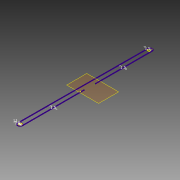
# Autodesk Inventor part: FDM20-BandaX-01
Saved by Autodesk Inventor 2015 (Build 190159000, 159)
## iProperties
Created: 2016-07-12
Part Number: FDM20-BandaX-01
Material: Generic
Document SubType Name: Modeling
Designer: Proyectil
Density: 1 g/cm^3
Appearance: Default
Author: Proyectil
Autodesk Inventor part; units mm, degrees
ref_plane "YZ Plane" through (0, 0, 0) normal (1, 0, 0) x (0, 1, 0)
ref_plane "XZ Plane" through (0, 0, 0) normal (0, 1, 0) x (-1, 0, 0)
ref_plane "XY Plane" through (0, 0, 0) normal (0, 0, 1) x (1, 0, 0)
ref_plane "Work Plane1" through (0.0298, -19.0597, 0) normal (0, 0, 1) x (1, -0.0002116, 0)
sketch "Sketch1" plane through (0.0298, -19.0597, 0) normal (0, 0, 1) x (1, -0.0002116, 0)
  circle A0 centre (-5.65, -140.7495) radius 4.3281 projected
  arc A1 (-12.6499, -140.717) -> (1.35, -140.7495) centre (-5.65, -140.7495) ccw
  arc A2 (2, 214.6005) -> (-10.9999, 214.6307) centre (-4.5, 214.6005) ccw
  line L0 (-12.6499, -140.717) -> (-10.9999, 214.6307)
  line L1 (1.35, -140.7495) -> (1.35, 11.2032)
  line L2 (2, 214.6005) -> (2, 37.9844)
  line L3 (0.5, 37.9844) -> (0.5, 214.6005)
  arc A3 (0.5, 214.6005) -> (-9.4999, 214.6237) centre (-4.5, 214.6005) ccw
  line L4 (-9.4999, 214.6237) -> (-11.1499, -140.724)
  line L5 (-0.15, 11.2032) -> (-0.15, -140.7495)
  arc A4 (-11.1499, -140.724) -> (-0.15, -140.7495) centre (-5.65, -140.7495) ccw
  line L6 (-0.15, 11.2032) -> (1.35, 11.2032)
  line L7 (0.5, 37.9844) -> (2, 37.9844)
  point P0 (-0.0338, 19.0597)
  dimension "d3" = 1.5
  dimension "d4" = 1.5
  dimension "d5" = 5.5
  dimension "d6" = 5
  constraints: 16 end point, 9 point on circle, 4 centre point, 4 tangent, 2 vertical, 1 coincident, 1 horizontal, 1 parallel, 1 point on line, 3 other
  measures "d3" distance between parallel lines of L2 L3
  measures "d4" distance between parallel lines of L1 L5
  measures "d5" radius of A4
  measures "d6" radius of A3
extrude "Extrusion1" add sketch "Sketch1" along normal mid plane 6 contours L0 A2 L2 L7 L3 A3 L4 A4 L5 L6 L1 A1
body "Solid1"
